Autodesk Inventor part; units mm, degrees
(part 2 of 2)
  line L262 (-15.2783, -21.3912) -> (-14.8544, -21.7008)
  line L263 (-14.8544, -21.7008) -> (-15.6184, -23.0086)
  line L264 (-15.6184, -23.0086) -> (-16.2916, -22.5169)
  line L265 (-17.1618, -21.8814) -> (-16.1485, -20.7557)
  line L266 (-16.1485, -20.7557) -> (-15.7246, -21.0653)
  line L267 (-15.7246, -21.0653) -> (-16.4886, -22.3731)
  line L268 (-16.4886, -22.3731) -> (-17.1618, -21.8814)
  line L269 (-21.4848, -17.4508) -> (-17.7983, -15.8261)
  line L270 (-17.7983, -15.8261) -> (-17.1214, -16.5585)
  line L271 (-17.1214, -16.5585) -> (-19.0307, -20.1059)
  line L272 (-19.0307, -20.1059) -> (-19.7034, -19.3781)
  line L273 (-19.7034, -19.3781) -> (-18.3694, -17.0141)
  line L274 (-18.3694, -17.0141) -> (-20.8288, -18.1605)
  line L275 (-20.8288, -18.1605) -> (-21.4848, -17.4508)
  spline S232 degree 2 poles (-22.8617, -11.8697) (-22.4369, -11.6174) (-21.7194, -11.3744) (-21.4145, -11.3981) knots 0 0 0 1 2 2 2
  spline S233 degree 2 poles (-21.4145, -11.3981) (-21.1138, -11.4206) (-20.6108, -11.7718) (-20.4059, -12.1169) knots 0 0 0 1 2 2 2
  spline S234 degree 2 poles (-20.4059, -12.1169) (-20.1993, -12.4647) (-20.1332, -13.0718) (-20.261, -13.3524) knots 0 0 0 1 2 2 2
  spline S235 degree 2 poles (-20.261, -13.3524) (-20.3862, -13.6314) (-20.9376, -14.142) (-21.3624, -14.3943) knots 0 0 0 1 2 2 2
  spline S236 degree 2 poles (-21.3624, -14.3943) (-21.7977, -14.6528) (-22.494, -14.8832) (-22.8084, -14.8616) knots 0 0 0 1 2 2 2
  spline S237 degree 2 poles (-22.8084, -14.8616) (-23.1176, -14.837) (-23.6185, -14.4773) (-23.8171, -14.1428) knots 0 0 0 1 2 2 2
  spline S238 degree 2 poles (-23.8171, -14.1428) (-24.0268, -13.7897) (-24.0844, -13.1848) (-23.9539, -12.9026) knots 0 0 0 1 2 2 2
  spline S239 degree 2 poles (-23.9539, -12.9026) (-23.8272, -12.6262) (-23.2731, -12.114) (-22.8617, -11.8697) knots 0 0 0 1 2 2 2
  spline S240 degree 2 poles (-22.3714, -12.6953) (-22.9793, -13.0563) (-23.3521, -13.5471) (-23.2118, -13.7833) knots 0 0 0 1 2 2 2
  spline S241 degree 2 poles (-23.2118, -13.7833) (-23.0715, -14.0196) (-22.4606, -13.9297) (-21.85, -13.5671) knots 0 0 0 1 2 2 2
  spline S242 degree 2 poles (-21.85, -13.5671) (-21.2501, -13.2108) (-20.8708, -12.7126) (-21.0111, -12.4764) knots 0 0 0 1 2 2 2
  spline S243 degree 2 poles (-21.0111, -12.4764) (-21.1499, -12.2428) (-21.7688, -12.3374) (-22.3714, -12.6953) knots 0 0 0 1 2 2 2
  line L276 (-22.4897, -7.9413) -> (-21.5191, -10.2629)
  line L277 (-21.5191, -10.2629) -> (-22.1316, -10.5189)
  line L278 (-22.1316, -10.5189) -> (-22.4412, -9.7783)
  line L279 (-22.4412, -9.7783) -> (-24.3014, -10.556)
  line L280 (-24.3014, -10.556) -> (-23.9917, -11.2966)
  line L281 (-23.9917, -11.2966) -> (-24.5643, -11.536)
  spline S244 degree 2 poles (-24.5643, -11.536) (-24.6322, -11.3736) (-24.8095, -11.0696) (-24.8956, -10.9918) knots 0 0 0 1 2 2 2
  spline S245 degree 2 poles (-24.8956, -10.9918) (-24.999, -10.9045) (-25.2422, -10.8589) (-25.3894, -10.9071) knots 0 0 0 1 2 2 2
  line L282 (-25.3894, -10.9071) -> (-25.711, -10.138)
  line L283 (-25.711, -10.138) -> (-22.7997, -8.9209)
  line L284 (-22.7997, -8.9209) -> (-23.1022, -8.1973)
  line L285 (-23.1022, -8.1973) -> (-22.4897, -7.9413)
  dimension "d145" = 47.625
  constraints: 1 centre point, 1 coincident, 1 other
  measures "d145" diameter of A0
extrude "Text" cut sketch "Sketch26" against normal blind 1.905
sketch "Sketch28" plane through (0, 0, 0) normal (0, -1, 0) x (1, 0, 0)
  line L0 (3.8128, -6.604) -> (-3.8128, -6.604)
  line L1 (-3.8128, -6.604) -> (-7.6256, 0)
  line L2 (-7.6256, 0) -> (-3.8128, 6.604)
  line L3 (-3.8128, 6.604) -> (3.8128, 6.604)
  line L4 (3.8128, 6.604) -> (7.6256, 0)
  line L5 (7.6256, 0) -> (3.8128, -6.604)
  line L6 (3.8128, -6.604) -> (-3.8128, -6.604) projected
  point P0 (0, 0)
  point P1 (0, 0)
  constraints: 12 end point, 1 coincident, 1 collinear, 1 horizontal, 13 other
extrude "Extrusion21" add sketch "Sketch28" against normal blind 76.2
sketch "Sketch29" plane through (0, 0, 0) normal (0, -1, 0) x (1, 0, 0)
  arc A0 (6.4104, 1.5875) -> (6.4104, -1.5875) centre (0, 0) ccw
  line L0 (0, 0) -> (6.604, 0) construction
  line L1 (6.4104, 1.5875) -> (5.0165, 1.5875)
  line L2 (5.0165, 1.5875) -> (5.0165, 0)
  line L3 (5.0165, 0) -> (5.0165, -1.5875)
  line L4 (5.0165, -1.5875) -> (6.4104, -1.5875)
  point P0 (5.7134, -1.5875)
  dimension "d161" = 13.208
  dimension "d162" = 1.5875
  dimension "d163" = 3.175
  constraints: 10 end point, 2 horizontal, 2 perpendicular, 2 point on circle, 2 point on line, 1 centre point, 1 coincident, 1 collinear, 1 midpoint
  measures "d161" diameter of A0
  measures "d162" distance of L0.end L2.end
  measures "d163" distance from line of point (5.713, -1.587) L1
extrude "Extrusion22" cut sketch "Sketch29" against normal through all
split "Split1" plane through (0, 38.1, 0) removes the side toward (0, 1, 0)
equation "\"d103\" = hexDiameter"
equation "\"d110\" = centerLineForSpool"
equation "\"d111\" = centerLineForSpool"
equation "\"d112\" = holeForString"
equation "\"d121\" = centerLineForSpool"
equation "\"d122\" = holeForString"
equation "\"d125\" = knotHoleDiameter"
equation "\"d127\" = holeForString"
equation "\"d128\" = centerLineForSpool"
equation "\"d129\" = knotHoleDiameter"
equation "\"d130\" = knotHoleDepth"
equation "\"d86\" = spoolOverallHeight"
equation "\"d89\" = 0.5 * spoolOverallHeight"
equation "\"centerLineForSpool\" = 0.25 * spoolOverallHeight"
equation "\"holeForString\" = stringDiameter + clearanceForString"
equation "\"stringDiameter\" = 3.048"
equation "\"clearanceForString\" = 2.032"
equation "\"hexShaftDiameter\" = 12.7"
equation "\"clearanceForHexShaft\" = 0.508"
equation "\"hexDiameter\" = hexShaftDiameter + clearanceForHexShaft"
equation "\"spoolInteriorDiameter\" = 38.1"
equation "\"spoolInteriroRadius\" = 0.5 * spoolInteriorDiameter"
equation "\"spoolExteriorDiameter\" = 63.5"
equation "\"spoolExteriorRadius\" = 0.5 * spoolExteriorDiameter"
equation "\"hexHoleChamfer\" = 1.5875"
equation "\"stringHoleCenterFromHexShaft\" = 0.5 * hexDiameter + 0.5 * holeForString"
equation "\"textCircleDiameter\" = 0.75 * spoolExteriorDiameter"
equation "\"textHeight\" = 4.572"
equation "\"textDepth\" = 1.27"
equation "\"spoolOverallHeight\" = 76.2"
equation "\"d114\" = -spoolInteriroRadius"
equation "\"knotHoleDiameter\" = 9.525"
equation "\"d126\" = spoolInteriroRadius"
equation "\"metalWasherID\" = 26.67"
equation "\"metalWasherThickness\" = 0"
equation "\"spacerOD\" = 24.13"
equation "\"spacerThickness\" = 2.54"
equation "\"knotHoleDepth\" = 11.1125"
body "Solid3"
